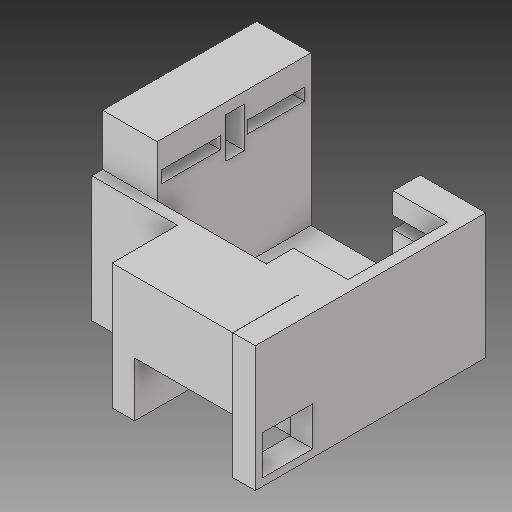
# Autodesk Inventor part: thingy_for_arms_servo
Saved by Autodesk Inventor 2018 (Build 220112000, 112)
## iProperties
Created: 2017-10-31
Part Number: thingy_for_arms_servo
Material: Generic
Document SubType Name: Modeling
Designer: khajemat000
Density: 1 g/cm^3
Appearance: Default
Author: khajemat000
Autodesk Inventor part; units mm, degrees
ref_plane "YZ Plane" through (0, 0, 0) normal (1, 0, 0) x (0, 1, 0)
ref_plane "XZ Plane" through (0, 0, 0) normal (0, 1, 0) x (-1, 0, 0)
ref_plane "XY Plane" through (0, 0, 0) normal (0, 0, 1) x (1, 0, 0)
sketch "Sketch1" plane through (0, 0, 0) normal (1, 0, 0) x (0, 1, 0)
  line L0 (0, 0) -> (22.86, 0)
  line L1 (22.86, 0) -> (22.86, -22.86)
  line L2 (22.86, -22.86) -> (0, -22.86)
  line L3 (0, -22.86) -> (0, 0)
  line L4 (0, -22.86) -> (15.24, -22.86)
  line L5 (0, -22.86) -> (15.24, -22.86) construction
  line L6 (15.24, -22.86) -> (15.24, -27.94)
  line L7 (15.24, -27.94) -> (17.78, -27.94)
  line L8 (17.78, -27.94) -> (17.78, -22.86)
  line L9 (17.78, 0) -> (17.78, 5.08)
  line L10 (17.78, 5.08) -> (15.24, 5.08)
  line L11 (15.24, 5.08) -> (15.24, 0)
  line L12 (17.9128, 0) -> (15.0818, 0)
  line L13 (15.0818, 5.3336) -> (17.9128, 5.3336)
  line L14 (17.9128, -22.86) -> (15.0818, -22.86)
  line L15 (15.0818, -28.1853) -> (17.9128, -28.1853)
  line L16 (17.9128, 0.0837) -> (17.9128, 5.3336)
  line L17 (15.0818, 0.0837) -> (15.0818, 5.3336)
  line L18 (15.0818, 0.0837) -> (-0.2071, 0.0837)
  line L19 (-0.2071, 0.0837) -> (-0.2071, -23.0588)
  line L20 (-0.2071, -23.0588) -> (15.0818, -23.0588)
  line L21 (15.0818, -23.0588) -> (15.0818, -28.1853)
  line L22 (17.9128, -28.1853) -> (17.9128, -23.0588)
  line L23 (17.9128, -23.0588) -> (22.86, -23.0588)
  line L24 (22.86, -23.0588) -> (22.86, -29.4177)
  line L25 (22.86, -29.4177) -> (-6.35, -29.4177)
  line L26 (22.86, 0.0837) -> (17.9128, 0.0837)
  line L27 (22.86, 0.0837) -> (22.86, 6.4337)
  line L28 (22.86, 6.4337) -> (-6.35, 6.4337)
  line L29 (-6.35, -29.4177) -> (-6.35, 6.4337)
  dimension "d0" = 22.86
  dimension "d1" = 22.86
  dimension "d4" = 5.08
  dimension "d5" = 2.54
  dimension "d6" = 5.08
  dimension "d7" = 2.54
  dimension "d9" = 29.21
  dimension "d11" = 6.35
  constraints: 60 end point, 9 perpendicular, 9 point on line, 6 parallel, 4 horizontal, 2 collinear, 1 vertical
  measures "d0" distance of L1.end L2.end
  measures "d1" distance of L0.end L1.end
  measures "d4" distance of L4.end L6.end
  measures "d5" distance of L6.end L7.end
  measures "d6" distance of L9.start L9.end
  measures "d7" distance of L9.end L10.end
  measures "d9" distance of L24.end L25.end
  measures "d11" distance of L26.start L27.end
extrude "Extrusion1" add sketch "Sketch1" along normal blind 12.7 contours L17 L18 L19 L20 L21 L15 L22 L23 L24 L25 L29 L28 L27 L26 L16 L13
sketch "Sketch2" plane through (12.7, 0, 0) normal (1, 0, 0) x (0, 0, -1)
  line L0 (-6.4337, 22.86) -> (-6.4337, -6.35) projected
  line L1 (29.4177, 22.86) -> (23.0588, 22.86) projected
  line L2 (-6.4337, -6.35) -> (29.4177, -6.35)
  line L3 (29.4177, -6.35) -> (29.4177, 22.86)
  line L4 (29.4177, 22.86) -> (-6.4337, 22.86)
  line L5 (-6.4337, 22.86) -> (-6.4337, -6.35)
  point P0 (0, 0)
  dimension "d16" = 29.21
  dimension "d17" = 35.8513
  constraints: 8 end point, 2 parallel, 1 horizontal, 1 perpendicular
  measures "d16" distance of L0.start L0.end
  measures "d17" distance of L0.end L2.end
extrude "Extrusion2" add sketch "Sketch2" along normal blind 2.54
sketch "Sketch3" plane through (0, 0, 0) normal (-1, 0, 0) x (0, 0, 1)
  line L0 (-29.4177, -6.35) -> (-29.4177, 22.86) projected
  line L1 (6.4337, -6.35) -> (-29.4177, -6.35) projected
  line L2 (-29.4177, 0) -> (6.4337, 0)
  line L3 (6.4337, 0) -> (6.4337, -6.35)
  line L4 (6.4337, -6.35) -> (-29.4177, -6.35)
  line L5 (-29.4177, -6.35) -> (-29.4177, 0)
  point P0 (0, 0)
  constraints: 8 end point, 2 parallel, 1 horizontal, 1 perpendicular, 1 point on line
extrude "Extrusion3" add sketch "Sketch3" along normal blind 25.4
sketch "Sketch4" plane through (-25.4, 0, 0) normal (-1, 0, 0) x (0, 0, 1)
  line L0 (6.4337, -6.35) -> (-29.4177, -6.35) projected
  line L1 (6.4337, 22.86) -> (6.4337, -6.35) projected
  line L2 (-29.4177, -6.35) -> (6.4337, -6.35)
  line L3 (6.4337, -6.35) -> (6.4337, 22.86)
  line L4 (-29.4177, 22.86) -> (-29.4177, -6.35)
  line L5 (6.4337, 32.258) -> (-29.4177, 32.258)
  line L6 (-29.4177, 32.258) -> (-29.4177, 22.86)
  line L7 (-29.4177, 32.258) -> (-7.1927, 32.258)
  line L8 (-7.1927, 32.258) -> (-11.6377, 32.258)
  line L9 (-29.4177, 22.86) -> (6.4337, 22.86) projected
  line L10 (-11.6377, 32.258) -> (-9.4152, 32.258)
  line L11 (-9.4152, 22.86) -> (-11.6377, 22.86)
  line L12 (-9.4152, 22.86) -> (-13.8602, 22.86)
  line L13 (-13.8602, 22.86) -> (-13.8602, 32.258)
  line L14 (-13.8602, 32.258) -> (-9.4152, 32.258)
  line L15 (-27.8895, 28.6463) -> (-14.6164, 28.6463)
  line L16 (-14.6164, 28.6463) -> (-14.6164, 25.8191)
  line L17 (-14.6164, 25.8191) -> (-27.8895, 25.8191)
  line L18 (-27.8895, 25.8191) -> (-27.8895, 28.6463)
  line L19 (-8.2851, 28.6463) -> (5.4248, 28.6463)
  line L20 (5.4248, 28.6463) -> (5.4248, 25.8191)
  line L21 (5.4248, 25.8191) -> (-8.2851, 25.8191)
  line L22 (-8.2851, 25.8191) -> (-8.2851, 28.6463)
  line L23 (-8.2851, 28.6463) -> (5.4248, 28.6463)
  line L24 (5.4248, 28.6463) -> (5.4248, 25.8191)
  line L25 (5.4248, 25.8191) -> (-8.2851, 25.8191)
  line L26 (-8.2851, 25.8191) -> (-8.2851, 28.6463)
  line L27 (6.4337, 32.258) -> (-9.4152, 32.258)
  line L28 (-9.4152, 32.258) -> (-9.4152, 22.86)
  line L29 (-9.4152, 22.86) -> (6.4337, 22.86)
  line L30 (6.4337, 22.86) -> (6.4337, 32.258)
  line L31 (-29.4177, -6.35) -> (-29.4177, 22.86) projected
  line L32 (0.0837, 22.86) -> (6.4337, 22.86) projected
  line L33 (-29.4177, 22.86) -> (6.4337, 22.86)
  line L34 (6.4337, 22.86) -> (6.4337, 32.258)
  line L35 (6.4337, 32.258) -> (-29.4177, 32.258)
  line L36 (-29.4177, 22.86) -> (-29.4177, 32.258)
  point P0 (0, 0)
  dimension "d21" = 22.225
  dimension "d23" = 2.2225
  dimension "d24" = 4.445
  constraints: 64 end point, 11 parallel, 7 horizontal, 7 perpendicular, 6 point on line, 3 collinear
  measures "d21" distance of L5.end L7.end
  measures "d23" distance of L11.start L11.end
  measures "d24" distance of L13.end L14.end
extrude "Extrusion7" add sketch "Sketch4" along normal blind 12.7 contours L0 L4 L9 L1 | L9 L28 L5 L30 | L6 L5 L13 L9
sketch "Sketch6" plane through (-25.4, 32.258, -13.8602) normal (0, 1, 0) x (1, 0, 0)
  line L0 (0, 15.5575) -> (-12.7, 15.5575) projected
  line L1 (0, -20.2938) -> (-12.7, -20.2938) projected
  line L2 (-12.7, 15.5575) -> (0, 15.5575)
  line L3 (0, 15.5575) -> (0, -20.2938)
  line L4 (0, -20.2938) -> (-12.7, -20.2938)
  line L5 (-12.7, -20.2938) -> (-12.7, 15.5575)
  point P0 (25.4, -13.8602)
  constraints: 8 end point, 2 parallel, 1 horizontal, 1 perpendicular
extrude "Extrusion8" add sketch "Sketch6" along normal blind 2.54
sketch "Sketch7" plane through (0, 22.86, 6.4337) normal (0, 0, 1) x (1, 0, 0)
  line L0 (0, 0) -> (15.24, 0) projected
  line L1 (-38.1, -29.21) -> (-38.1, 11.938) projected
  line L2 (15.24, 0) -> (-38.1, 0)
  line L3 (-38.1, 0) -> (-38.1, -29.21)
  line L4 (-38.1, -29.21) -> (15.24, -29.21)
  line L5 (15.24, -29.21) -> (15.24, 0)
  point P0 (0, -22.86)
  constraints: 8 end point, 2 parallel, 1 horizontal, 1 perpendicular
extrude "Extrusion9" add sketch "Sketch7" along normal blind 2.54
sketch "Sketch8" plane through (0, 22.86, -23.0588) normal (0, 1, 0) x (1, 0, 0)
  line L0 (15.24, -32.0324) -> (-38.1, -32.0324) projected
  line L1 (-12.8761, -32.0324) -> (9.9839, -32.0324)
  line L2 (-12.8761, -47.2724) -> (-12.8761, -32.0324)
  line L3 (9.9839, -47.2724) -> (15.24, -47.2724)
  line L4 (15.24, -32.0324) -> (9.9839, -32.0324)
  line L5 (9.9839, -32.0324) -> (9.9839, -47.2724)
  line L6 (-12.8761, -47.2724) -> (-18.1339, -47.2724)
  line L7 (-18.1339, -32.0324) -> (-12.8761, -32.0324)
  line L8 (-12.8761, -32.0324) -> (-12.8761, -47.2724)
  line L9 (9.9839, -32.0324) -> (15.24, -32.0324)
  line L10 (15.24, -47.2724) -> (9.9839, -47.2724)
  line L11 (9.9839, -47.2724) -> (9.9839, -32.0324)
  line L12 (-18.1339, -32.0324) -> (15.24, -32.0324)
  line L13 (15.24, -32.0324) -> (15.24, -47.2724)
  line L14 (15.24, -32.0324) -> (9.9839, -32.0324)
  line L15 (-18.1339, -47.2724) -> (-18.1339, -32.0324)
  line L16 (-12.8761, -32.0324) -> (-18.1339, -32.0324)
  point P0 (0, -23.0588)
  dimension "d37" = 22.86
  dimension "d39" = 5.2578
  constraints: 32 end point, 5 horizontal, 3 parallel, 2 collinear, 2 perpendicular, 2 point on line
  measures "d37" distance of L3.start L2.start
  measures "d39" distance of L7.start L7.end
extrude "Extrusion11" add sketch "Sketch8" against normal blind 29.21
sketch "Sketch9" plane through (-18.1339, 22.86, 24.2137) normal (0, 0, 1) x (1, 0, 0)
  line L0 (5.2578, -29.21) -> (0, -29.21) projected
  line L1 (5.2578, 0) -> (5.2578, -29.21) projected
  line L2 (5.2578, -16.51) -> (28.0868, -16.51)
  line L3 (28.0868, -16.51) -> (28.0868, 0)
  line L4 (28.0868, 0) -> (5.2578, 0)
  line L5 (5.2578, 0) -> (5.2578, -16.51)
  point P0 (18.1339, -22.86)
  dimension "d44" = 12.7
  constraints: 8 end point, 2 parallel, 1 horizontal, 1 perpendicular, 1 point on line
  measures "d44" distance of L0.start L2.start
extrude "Extrusion12" add sketch "Sketch9" against normal blind 15.5575
sketch "Sketch10" plane through (9.9839, 22.86, 8.9737) normal (-1, 0, 0) x (0, 0, 1)
  line L0 (1.8867, -18.3591) -> (13.634, -18.3591)
  line L1 (13.634, -18.3591) -> (13.634, -27.4569)
  line L2 (13.634, -27.4569) -> (1.8867, -27.4569)
  line L3 (1.8867, -27.4569) -> (1.8867, -18.3591)
  point P0 (-8.9737, -22.86)
  constraints: 8 end point, 2 parallel, 1 horizontal, 1 perpendicular
extrude "Extrusion13" cut sketch "Sketch10" against normal blind 15.5575
sketch "Sketch11" plane through (15.24, 22.86, -29.4177) normal (0, 0, -1) x (-1, 0, 0)
  line L0 (3.4492, -12.7029) -> (13.9615, -12.7029)
  line L1 (13.9615, -12.7029) -> (13.9615, -21.6525)
  line L2 (13.9615, -21.6525) -> (3.4492, -21.6525)
  line L3 (3.4492, -21.6525) -> (3.4492, -12.7029)
  point P0 (15.24, -22.86)
  constraints: 8 end point, 2 parallel, 1 horizontal, 1 perpendicular
extrude "Extrusion14" cut sketch "Sketch11" against normal blind 15.5575
body "Solid1"
